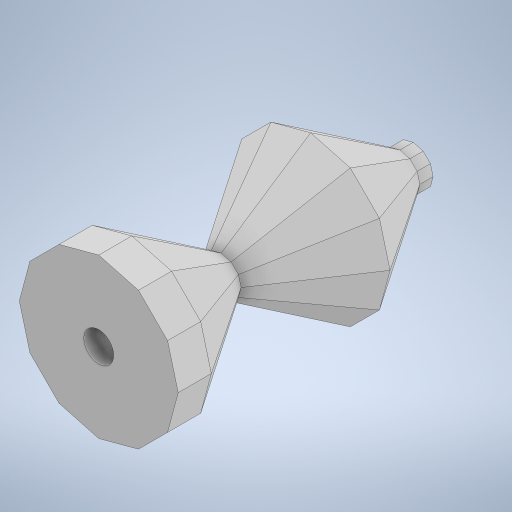
# Autodesk Inventor part: Test27
Saved by Autodesk Inventor 2023 (Build 270158000, 158)
## iProperties
Created: 2024-07-02
Part Number: Test27
Material: 일반
Document SubType Name: Modeling
Designer: ojs08
Density: 1 g/cm^3
Appearance: 기본값
Author: ojs08
Autodesk Inventor part; units mm, degrees
ref_plane "YZ Plane" through (0, 0, 0) normal (1, 0, 0) x (0, 1, 0)
ref_plane "XZ Plane" through (0, 0, 0) normal (0, 1, 0) x (-1, 0, 0)
sketch "스케치1" plane through (0, 0, 0) normal (0, 0, 1) x (1, 0, 0)
  line L0 (10.3923, 6) -> (12, 0)
  line L1 (12, 0) -> (10.3923, -6)
  line L2 (10.3923, -6) -> (6, -10.3923)
  line L3 (6, -10.3923) -> (0, -12)
  line L4 (0, -12) -> (-6, -10.3923)
  line L5 (-6, -10.3923) -> (-10.3923, -6)
  line L6 (-10.3923, -6) -> (-12, 0)
  line L7 (-12, 0) -> (-10.3923, 6)
  line L8 (-10.3923, 6) -> (-6, 10.3923)
  line L9 (-6, 10.3923) -> (0, 12)
  line L10 (0, 12) -> (6, 10.3923)
  line L11 (6, 10.3923) -> (10.3923, 6)
  line L12 (-16.8, 0) -> (16.8, 0) projected
  point P0 (0, 0)
  point P1 (0, 0)
  dimension "d0" = 24
  constraints: 24 end point, 1 coincident, 1 point on line, 25 other
  measures "d0" distance of L0.end L6.end
ref_plane "작업 평면1" through (0, 0, 13.5) normal (0, 0, 1) x (1, 0, 0)
sketch "스케치2" plane through (0, 0, 13.5) normal (0, 0, 1) x (1, 0, 0)
  line L0 (2.5981, 1.5) -> (3, 0)
  line L1 (3, 0) -> (2.5981, -1.5)
  line L2 (2.5981, -1.5) -> (1.5, -2.5981)
  line L3 (1.5, -2.5981) -> (0, -3)
  line L4 (0, -3) -> (-1.5, -2.5981)
  line L5 (-1.5, -2.5981) -> (-2.5981, -1.5)
  line L6 (-2.5981, -1.5) -> (-3, 0)
  line L7 (-3, 0) -> (-2.5981, 1.5)
  line L8 (-2.5981, 1.5) -> (-1.5, 2.5981)
  line L9 (-1.5, 2.5981) -> (0, 3)
  line L10 (0, 3) -> (1.5, 2.5981)
  line L11 (1.5, 2.5981) -> (2.5981, 1.5)
  line L12 (-4.2, 0) -> (4.2, 0) projected
  point P0 (0, 0)
  point P1 (0, 0)
  dimension "d2" = 6
  constraints: 24 end point, 1 coincident, 1 point on line, 25 other
  measures "d2" distance of L0.end L6.end
loft "로프트1" add profiles "스케치1", "스케치2"
mirror "미러1" about plane through (0, 0, 13.5) normal (0, 0, 1) of "로프트1"
mirror "미러2" about plane through (0, 0, 0) normal (0, 0, -1) of "로프트1"
sketch "스케치3" plane through (12, 0, 27) normal (0, 0, 1) x (0.9659258, 0.258819, 0)
  line L0 (0, 6.2117) -> (0, 0) projected
  line L1 (-3.1058, 11.5911) -> (0, 6.2117) projected
  line L2 (-8.4853, 14.6969) -> (-3.1058, 11.5911) projected
  line L3 (-14.6969, 14.6969) -> (-8.4853, 14.6969) projected
  line L4 (-20.0764, 11.5911) -> (-14.6969, 14.6969) projected
  line L5 (-23.1822, 6.2117) -> (-20.0764, 11.5911) projected
  line L6 (-23.1822, 0) -> (-23.1822, 6.2117) projected
  line L7 (-20.0764, -5.3795) -> (-23.1822, 0) projected
  line L8 (-14.6969, -8.4853) -> (-20.0764, -5.3795) projected
  line L9 (-8.4853, -8.4853) -> (-14.6969, -8.4853) projected
  line L10 (-3.1058, -5.3795) -> (-8.4853, -8.4853) projected
  line L11 (0, 0) -> (-3.1058, -5.3795) projected
  point P0 (-11.5911, 3.1058)
extrude "돌출1" add sketch "스케치3" along normal blind 2
shell "쉘1" thickness 0.5 removed faces 0 ; own thickness 2 on faces at (-7.1716, -7.1716, -2.25) (-9.7966, -2.625, -2.25) (-9.7966, 2.625, -2.25) (-7.1716, 7.1716, -2.25) (-2.625, 9.7966, -2.25) (2.625, 9.7966, -2.25) (-2.625, -9.7966, -2.25) (2.625, -9.7966, -2.25) (7.1716, -7.1716, -2.25) (9.7966, -2.625, -2.25) (9.7966, 2.625, -2.25) (7.1716, 7.1716, -2.25) (-7.1716, 7.1716, 24.75) (-2.625, 9.7966, 24.75) (2.625, 9.7966, 24.75) (7.1716, 7.1716, 24.75) (9.7966, 2.625, 24.75) (9.7966, -2.625, 24.75) (7.1716, -7.1716, 24.75) (2.625, -9.7966, 24.75) (-2.625, -9.7966, 24.75) (-7.1716, -7.1716, 24.75) (-9.7966, 2.625, 24.75) (-9.7966, -2.625, 24.75)
sketch "스케치4" plane through (12, 0, 29) normal (0, 0, 1) x (0.9659258, 0.258819, 0)
  line L0 (-3.1058, 11.5911) -> (-8.4853, 14.6969) projected
  line L1 (-8.4853, 14.6969) -> (-14.6969, 14.6969) projected
  line L2 (-14.6969, 14.6969) -> (-20.0764, 11.5911) projected
  line L3 (-20.0764, 11.5911) -> (-23.1822, 6.2117) projected
  line L4 (-23.1822, 6.2117) -> (-23.1822, 0) projected
  line L5 (-23.1822, 0) -> (-20.0764, -5.3795) projected
  line L6 (-20.0764, -5.3795) -> (-14.6969, -8.4853) projected
  line L7 (-14.6969, -8.4853) -> (-8.4853, -8.4853) projected
  line L8 (-8.4853, -8.4853) -> (-3.1058, -5.3795) projected
  line L9 (-3.1058, -5.3795) -> (0, 0) projected
  line L10 (0, 0) -> (0, 6.2117) projected
  line L11 (0, 6.2117) -> (-3.1058, 11.5911) projected
  point P0 (-11.5911, 3.1058)
extrude "돌출2" add sketch "스케치4" along normal blind 3
sketch "스케치5" plane through (12, 0, 32) normal (0, 0, 1) x (0.9659258, 0.258819, 0)
  circle A0 centre (-11.5911, 3.1058) radius 2.25
  dimension "d13" = 4.5
  constraints: 1 centre point, 1 coincident
  measures "d13" diameter of A0
extrude "돌출3" cut sketch "스케치5" against normal blind 5
sketch "스케치6" plane through (3, 0, -13.5) normal (0, 0, -1) x (-0.9659258, -0.258819, 0)
  line L0 (0, 1.5529) -> (0, 0) projected
  line L1 (0, 0) -> (0.7765, -1.3449) projected
  line L2 (0.7765, -1.3449) -> (2.1213, -2.1213) projected
  line L3 (2.1213, -2.1213) -> (3.6742, -2.1213) projected
  line L4 (3.6742, -2.1213) -> (5.0191, -1.3449) projected
  line L5 (5.0191, -1.3449) -> (5.7956, 0) projected
  line L6 (5.7956, 0) -> (5.7956, 1.5529) projected
  line L7 (5.7956, 1.5529) -> (5.0191, 2.8978) projected
  line L8 (5.0191, 2.8978) -> (3.6742, 3.6742) projected
  line L9 (3.6742, 3.6742) -> (2.1213, 3.6742) projected
  line L10 (2.1213, 3.6742) -> (0.7765, 2.8978) projected
  line L11 (0.7765, 2.8978) -> (0, 1.5529) projected
  point P0 (2.8978, 0.7765)
extrude "돌출4" add sketch "스케치6" along normal blind 2
